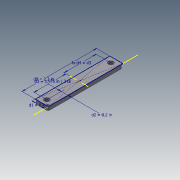
# Autodesk Inventor part: Standard
Saved by Autodesk Inventor 2020.3 (Build 243373000, 373)
## iProperties
RuleStatus: InUse
AfterDocSave0: file://Part Number Cleaner
Created: 2023-02-10
Material: Generic
Catalog Web Link: https://www.janelia.org/
Vendor: HHMI: JRC - jET
Document SubType Name: Modeling
Designer: arnoldj
Density: 1 g/cm^3
Appearance: Default
DESIGN DEPARTMENT: HHMI: JRC - jET
ALTERED ITEM PART NUMBER: N/A
ALTERED ITEM VENDOR: N/A
ALTERED ITEM DESCRIPTION: N/A
Title: Standard
Author: arnoldj
Revision Number: 0
Autodesk Inventor part; units mm, degrees
ref_plane "YZ Plane" through (0, 0, 0) normal (1, 0, 0) x (0, 1, 0)
ref_plane "XZ Plane" through (0, 0, 0) normal (0, 1, 0) x (-1, 0, 0)
ref_plane "XY Plane" through (0, 0, 0) normal (0, 0, 1) x (1, 0, 0)
sketch "Sketch1" plane through (0, 0, 0) normal (0, 1, 0) x (-1, 0, 0)
  line L0 (-2.032, 0) -> (12.192, 0) projected
  line L1 (0, -40.894) -> (0, 40.894) projected
  line L2 (10.16, -29.21) -> (0, -29.21)
  line L3 (0, -29.21) -> (0, 29.21)
  line L4 (0, 29.21) -> (10.16, 29.21)
  line L5 (10.16, 29.21) -> (10.16, -29.21)
  line L6 (10.16, -29.21) -> (0, 29.21) construction
  line L7 (0, -29.21) -> (10.16, 29.21) construction
  point P0 (0, 0)
  point P1 (5.08, 0)
  point P2 (5.08, 25.0825)
  point P3 (5.08, 0)
  point P4 (5.08, -25.0825)
  point P5 (0, -29.21)
  dimension "d0" = 58.42
  dimension "d1" = 10.16
  dimension "d2" = 5.08
  dimension "d3" = 25.0825
  dimension "d4" = 25.0825
  constraints: 12 end point, 4 midpoint, 2 parallel, 2 vertical alignment, 1 horizontal, 1 perpendicular, 1 point on line
  measures "d0" distance of L4.end L2.start
  measures "d1" distance of L3.end L4.end
  measures "d2" distance from line of point (5.08, 25.083) L3
  measures "d3" distance from line of L0 point (5.08, 25.083)
  measures "d4" distance from line of point (5.08, -25.083) L0
extrude "Extrusion1" add sketch "Sketch1" against normal blind 3.175
fillet "Fillet1" radius 1.27 2 edges at (-10.16, -1.5875, 29.21) (-10.16, -1.5875, -29.21)
fillet "Fillet2" radius 1.27 2 edges at (0, -1.5875, 29.21) (0, -1.5875, -29.21)
hole "Hole1" at (-5.08, 0, 25.0825) at (-5.08, 0, -25.0825) direction (0, -1, 0) diameter 4.064 end through all
equation "\"d4\" = d3"
body "Solid1"
